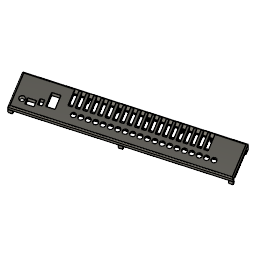
HV Interlock panel (Autodesk Fusion 360 design; units mm, degrees)
Autodesk Fusion 360 part; units mm, degrees
sketch "Sketch1" plane through (0, 0, 0) normal (0, 0, 1) x (1, 0, 0)
  line L0 (152.4, -27.305) -> (-152.4, -27.305)
  line L1 (-152.4, -27.305) -> (-152.4, 27.305)
  line L2 (-152.4, 27.305) -> (152.4, 27.305)
  line L3 (152.4, 27.305) -> (152.4, -27.305)
  line L4 (152.4, -27.305) -> (-152.4, 27.305) construction
  line L5 (-152.4, -27.305) -> (152.4, 27.305) construction
  dimension "d1" = 304.8
  dimension "d2" = 54.61
  constraint horizontal L0
  constraint perpendicular L0 L1
  constraint parallel L0 L2
  constraint parallel L1 L3
  constraint coincident L4 origin
  constraint coincident L5 origin
  measures "d1" distance of L1.end L2.end
  measures "d2" distance of L0.end L1.end
extrude "Extrude1" add sketch "Sketch1" along normal blind 8.001 makes body 1
sketch "Sketch2" plane through (0, 0, 0) normal (0, 0, -1) x (1, 0, 0)
  line L0 (-152.4, -27.305) -> (152.4, -27.305)
  line L1 (152.4, -27.305) -> (152.4, 27.305)
  line L2 (152.4, 27.305) -> (-152.4, 27.305)
  line L3 (-152.4, 27.305) -> (-152.4, -27.305)
  line L4 (152.4, -22.225) -> (-152.4, -22.225)
  line L5 (-152.4, -22.225) -> (-152.4, 22.225)
  line L6 (-152.4, 22.225) -> (152.4, 22.225)
  line L7 (152.4, 22.225) -> (152.4, -22.225)
  line L8 (152.4, -22.225) -> (-152.4, 22.225) construction
  line L9 (-152.4, -22.225) -> (152.4, 22.225) construction
  line L10 (-152.4, 27.305) -> (-146.05, 27.305)
  line L11 (-146.05, 27.305) -> (-146.05, 19.685)
  line L12 (-146.05, 19.685) -> (-152.4, 19.685)
  line L13 (-152.4, 19.685) -> (-152.4, 27.305)
  dimension "d5" = 304.8
  dimension "d6" = 44.45
  dimension "d7" = 6.35
  dimension "d8" = 7.62
  constraint horizontal L4
  constraint perpendicular L4 L5
  constraint parallel L4 L6
  constraint parallel L5 L7
  constraint coincident L8 origin
  constraint coincident L9 origin
  constraint horizontal L10
  constraint vertical L11
  constraint horizontal L12
  constraint vertical L13
  constraint coincident L2.end L3.start
  measures "d5" distance of L5.end L6.end
  measures "d6" distance of L4.end L5.end
  measures "d7" distance of L2.end L10.end
  measures "d8" distance of L2.end L12.end
extrude "Extrude2" add sketch "Sketch2" along normal blind 7.874 contours L3 L5 L6 L11 L12 L13 | L2 L3 L6 L10 L11 L13 bodies 1
pattern_linear "R-Pattern1" count 8 spacing 42.6357 along (1, 0, 0) of "Extrude2"
sketch "Sketch3" plane through (152.4, 0, 0) normal (1, 0, 0) x (0, 1, 0)
  line L0 (-19.685, 0) -> (27.305, 0)
  line L1 (27.305, 0) -> (27.305, 8.001)
  line L2 (27.305, 8.001) -> (-27.305, 8.001)
  line L3 (-27.305, 8.001) -> (-27.305, -7.874)
  line L4 (-27.305, -7.874) -> (-19.685, -7.874)
  line L5 (-19.685, -7.874) -> (-19.685, 0)
  line L6 (-19.685, 0) -> (-22.225, 0)
  line L7 (-22.225, 0) -> (-22.225, -1.6256)
  line L8 (-22.225, -1.6256) -> (-19.685, -1.6256)
  line L9 (-19.685, -1.6256) -> (-19.685, 0)
  dimension "d15" = 2.54
  dimension "d16" = 1.6256
  constraint horizontal L6
  constraint vertical L7
  constraint horizontal L8
  constraint vertical L9
  constraint coincident L0.start L5.end
  measures "d15" distance of L0.start L6.end
  measures "d16" distance of L0.start L8.end
extrude "Extrude3" cut sketch "Sketch3" against normal blind 358.14 contours L5 L6 L7 L8 L9 bodies 1
sketch "Sketch4" plane through (0, 0, 0) normal (0, 0, -1) x (1, 0, 0)
  line L0 (146.05, 22.225) -> (146.05, 27.305)
  line L1 (146.05, 27.305) -> (109.7643, 27.305)
  line L2 (109.7643, 27.305) -> (109.7643, 22.225)
  line L3 (109.7643, 22.225) -> (103.4143, 22.225)
  line L4 (103.4143, 22.225) -> (103.4143, 27.305)
  line L5 (103.4143, 27.305) -> (67.1286, 27.305)
  line L6 (67.1286, 27.305) -> (67.1286, 22.225)
  line L7 (67.1286, 22.225) -> (60.7786, 22.225)
  line L8 (60.7786, 22.225) -> (60.7786, 27.305)
  line L9 (60.7786, 27.305) -> (24.4929, 27.305)
  line L10 (24.4929, 27.305) -> (24.4929, 22.225)
  line L11 (24.4929, 22.225) -> (18.1429, 22.225)
  line L12 (18.1429, 22.225) -> (18.1429, 27.305)
  line L13 (18.1429, 27.305) -> (-18.1429, 27.305)
  line L14 (-18.1429, 27.305) -> (-18.1429, 22.225)
  line L15 (-18.1429, 22.225) -> (-24.4929, 22.225)
  line L16 (-24.4929, 22.225) -> (-24.4929, 27.305)
  line L17 (-24.4929, 27.305) -> (-60.7786, 27.305)
  line L18 (-60.7786, 27.305) -> (-60.7786, 22.225)
  line L19 (-60.7786, 22.225) -> (-67.1286, 22.225)
  line L20 (-67.1286, 22.225) -> (-67.1286, 27.305)
  line L21 (-67.1286, 27.305) -> (-103.4143, 27.305)
  line L22 (-103.4143, 27.305) -> (-103.4143, 22.225)
  line L23 (-103.4143, 22.225) -> (-109.7643, 22.225)
  line L24 (-109.7643, 22.225) -> (-109.7643, 27.305)
  line L25 (-109.7643, 27.305) -> (-146.05, 27.305)
  line L26 (-146.05, 27.305) -> (-146.05, 22.225)
  line L27 (-146.05, 22.225) -> (-152.4, 22.225)
  line L28 (-152.4, 22.225) -> (-152.4, -27.305)
  line L29 (-152.4, -27.305) -> (152.4, -27.305)
  line L30 (152.4, -27.305) -> (152.4, 22.225)
  line L31 (152.4, 22.225) -> (146.05, 22.225)
  line L32 (-152.4, -27.305) -> (-146.05, -27.305)
  line L33 (-146.05, -27.305) -> (-146.05, -22.098)
  line L34 (-146.05, -22.098) -> (-152.4, -22.098)
  line L35 (-152.4, -22.098) -> (-152.4, -27.305)
  dimension "d19" = 6.35
  dimension "d20" = 5.207
  constraint horizontal L32
  constraint vertical L33
  constraint horizontal L34
  constraint vertical L35
  constraint coincident L28.end L29.start
  measures "d19" distance of L28.end L32.end
  measures "d20" distance of L28.end L34.end
extrude "Extrude4" add sketch "Sketch4" along normal up to surface (7.874 mm away) separate body contours L28 L29 L32 L33 L34 L35 makes body 2
pattern_linear "R-Pattern2" count 3 spacing 149.225 along (1, 0, 0) of "Extrude4" makes body 3 makes body 4
sketch "Sketch5" plane through (-152.4, 0, 0) normal (-1, 0, 0) x (0, -1, 0)
  line L0 (-27.305, -7.874) -> (-22.098, -7.874)
  line L1 (-22.098, -7.874) -> (-22.098, 0)
  line L2 (-22.098, 0) -> (-27.305, 0)
  line L3 (-27.305, 0) -> (-27.305, -7.874)
  line L4 (-24.638, 0) -> (-24.638, -1.524)
  line L5 (-24.638, -1.524) -> (-22.098, -3.937)
  line L6 (-22.098, -3.937) -> (-24.7015, -7.874)
  line L7 (-24.7015, -7.874) -> (-22.098, -7.874)
  line L8 (-22.098, -7.874) -> (-22.098, 0)
  line L9 (-22.098, 0) -> (-24.638, 0)
  point P0 (-24.638, 0)
  dimension "d27" = 2.54
  dimension "d28" = 1.524
  constraint coincident L2 P0
  constraint coincident P0 L4.start
  constraint perpendicular L2 L4
  constraint midpoint L1 L5.end
  constraint midpoint L0 L6.end
  constraint coincident L0.end L1.start
  constraint coincident L1.end L2.start
  measures "d27" distance of L1 P0
  measures "d28" distance of P0 L4.end
extrude "Extrude5" cut sketch "Sketch5" against normal blind 358.14 contours L0 L1 L6 L7 L8 | L1 L2 L4 L5 L8 L9 bodies 2 3 4
sketch "Sketch6" plane through (-152.4, 0, 0) normal (-1, 0, 0) x (0, -1, 0)
  line L0 (22.225, -1.6256) -> (19.685, -1.6256)
  line L1 (19.685, -1.6256) -> (19.685, -7.874)
  line L2 (19.685, -7.874) -> (27.305, -7.874)
  line L3 (27.305, -7.874) -> (27.305, 8.001)
  line L4 (27.305, 8.001) -> (-27.305, 8.001)
  line L5 (-27.305, 8.001) -> (-27.305, 0)
  line L6 (-27.305, 0) -> (22.225, 0)
  line L7 (22.225, 0) -> (22.225, -1.6256)
  line L8 (-24.6876, 0) -> (-24.6876, 4.0005)
  line L9 (-24.6876, 4.0005) -> (-21.59, 4.0005)
  line L10 (-21.59, 4.0005) -> (-21.59, 0)
  line L11 (-21.59, 0) -> (-24.6876, 0)
  constraint coincident L6 L8.start
  constraint perpendicular L4 L8
  constraint perpendicular L8 L9
  constraint coincident L6 L10.end
  constraint perpendicular L6 L10
extrude "Extrude6" cut sketch "Sketch6" against normal blind 320.04 contours L6 L8 L9 L10 L11 bodies 1
fillet "Fillet1" radius 1.27 1 edges at (0, 24.6876, 4.0005) on bodies 1
sketch "Sketch8" plane through (0, 0, 8.001) normal (0, 0, 1) x (-1, 0, 0)
  line L0 (-152.4, -27.305) -> (152.4, -27.305)
  line L1 (152.4, -27.305) -> (152.4, 27.305)
  line L2 (152.4, 27.305) -> (-152.4, 27.305)
  line L3 (-152.4, 27.305) -> (-152.4, -27.305)
  line L4 (2.794, 5.715) -> (-2.794, 5.715)
  line L5 (-2.794, 5.715) -> (-2.794, 20.955)
  line L6 (-2.794, 20.955) -> (2.794, 20.955)
  line L7 (2.794, 20.955) -> (2.794, 5.715)
  line L8 (2.794, 5.715) -> (-2.794, 20.955) construction
  line L9 (-2.794, 5.715) -> (2.794, 20.955) construction
  point P0 (0, 13.335)
  dimension "d35" = 5.588
  dimension "d36" = 15.24
  dimension "d37" = 13.97
  constraint horizontal L4
  constraint perpendicular L4 L5
  constraint parallel L4 L6
  constraint parallel L5 L7
  constraint coincident L8 P0
  constraint coincident L9 P0
  measures "d35" distance of L5.end L6.end
  measures "d36" distance of L4.end L5.end
  measures "d37" distance of L2 P0
sketch "PCB" plane through (0, 0, 8.001) normal (0, 0, 1) x (-1, 0, 0)
  line L0 (-152.4, -27.305) -> (152.4, -27.305)
  line L1 (152.4, -27.305) -> (152.4, 27.305)
  line L2 (152.4, 27.305) -> (-152.4, 27.305)
  line L3 (-152.4, 27.305) -> (-152.4, -27.305)
  circle A0 centre (-32.5558, -7.8785) radius 0.85
  circle A1 centre (-37.4758, -7.8785) radius 0.85
  circle A2 centre (-139.3358, -10.4185) radius 0.6
  circle A3 centre (32.5242, -7.8785) radius 0.85
  circle A4 centre (22.5242, -7.8785) radius 0.85
  circle A5 centre (-136.7958, -7.8785) radius 0.85
  circle A6 centre (-100.0708, 3.8415) radius 0.5
  circle A7 centre (27.4442, -12.9585) radius 0.85
  circle A8 centre (29.9842, -10.4185) radius 0.6
  circle A9 centre (-129.8408, -10.4185) radius 0.5
  circle A10 centre (-102.6108, 3.8415) radius 0.5
  circle A11 centre (17.4442, -12.9585) radius 0.85
  circle A12 centre (-141.8758, -7.8785) radius 0.85
  circle A13 centre (42.5242, -7.8785) radius 0.85
  circle A14 centre (-27.4758, -7.8785) radius 0.85
  circle A15 centre (19.9842, -10.4185) radius 0.6
  circle A16 centre (-113.6508, -4.6785) radius 0.5
  circle A17 centre (-222.1058, -16.0685) radius 3.2
  circle A18 centre (37.4442, -7.8785) radius 0.85
  circle A19 centre (-141.8758, -12.9585) radius 0.85
  circle A20 centre (-42.5558, -7.8785) radius 0.85
  circle A21 centre (-124.6058, -12.9585) radius 0.5
  circle A22 centre (-129.8408, -12.9585) radius 0.5
  circle A23 centre (-124.6058, -10.4185) radius 0.5
  circle A24 centre (-40.0158, -10.4185) radius 0.6
  circle A25 centre (-30.0158, -10.4185) radius 0.6
  circle A26 centre (-42.5558, -12.9585) radius 0.85
  circle A27 centre (-37.4758, -12.9585) radius 0.85
  circle A28 centre (39.9842, -10.4185) radius 0.6
  circle A29 centre (-136.7958, -12.9585) radius 0.85
  circle A30 centre (27.4442, -7.8785) radius 0.85
  circle A31 centre (-103.6256, -4.568) radius 0.7
  circle A32 centre (-78.4158, 15.6015) radius 0.5
  circle A33 centre (-116.1908, -4.6785) radius 0.5
  circle A34 centre (-98.5456, -4.568) radius 0.7
  circle A35 centre (-32.5558, -12.9585) radius 0.85
  circle A36 centre (-49.9558, -10.4185) radius 0.6
  circle A37 centre (-58.4158, 10.6015) radius 0.5
  circle A38 centre (-68.4158, 13.1015) radius 0.5
  circle A39 centre (-68.4158, 10.6015) radius 0.5
  circle A40 centre (-57.4758, -7.8785) radius 0.85
  circle A41 centre (-68.4158, 15.6015) radius 0.5
  circle A42 centre (-67.4758, -7.8785) radius 0.85
  circle A43 centre (-72.5558, -7.8785) radius 0.85
  circle A44 centre (-47.4158, -7.8785) radius 0.85
  circle A45 centre (-58.4158, 15.6015) radius 0.5
  circle A46 centre (-52.4958, -7.8785) radius 0.85
  circle A47 centre (-78.4158, 13.1015) radius 0.5
  circle A48 centre (-70.0158, -10.4185) radius 0.6
  circle A49 centre (-67.4758, -12.9585) radius 0.85
  circle A50 centre (-57.4758, -12.9585) radius 0.85
  circle A51 centre (-48.4158, 10.6015) radius 0.5
  circle A52 centre (-27.4758, -12.9585) radius 0.85
  circle A53 centre (-48.4158, 15.6015) radius 0.5
  circle A54 centre (-78.4158, 10.6015) radius 0.5
  circle A55 centre (-58.4158, 13.1015) radius 0.5
  circle A56 centre (-62.5558, -7.8785) radius 0.85
  circle A57 centre (-48.4158, 13.1015) radius 0.5
  circle A58 centre (-60.0158, -10.4185) radius 0.6
  circle A59 centre (-72.5558, -12.9585) radius 0.85
  circle A60 centre (-62.5558, -12.9585) radius 0.85
  circle A61 centre (-47.4158, -12.9585) radius 0.85
  circle A62 centre (-52.4958, -12.9585) radius 0.85
  circle A63 centre (-10.0158, -10.4185) radius 0.6
  circle A64 centre (17.4442, -7.8785) radius 0.85
  circle A65 centre (-7.4758, -7.8785) radius 0.85
  circle A66 centre (-17.4758, -7.8785) radius 0.85
  line L4 (-230.9558, 22.6815) -> (-230.9558, -21.7685)
  circle A67 centre (-20.0158, -10.4185) radius 0.6
  circle A68 centre (32.5242, -12.9585) radius 0.85
  circle A69 centre (-7.4758, -12.9585) radius 0.85
  circle A70 centre (-12.5558, -12.9585) radius 0.85
  circle A71 centre (42.5242, -12.9585) radius 0.85
  circle A72 centre (-22.5558, -12.9585) radius 0.85
  circle A73 centre (37.4442, -12.9585) radius 0.85
  circle A74 centre (22.5242, -12.9585) radius 0.85
  circle A75 centre (-17.4758, -12.9585) radius 0.85
  circle A76 centre (97.4442, -7.8785) radius 0.85
  circle A77 centre (7.4442, -7.8785) radius 0.85
  circle A78 centre (-18.4158, 10.6015) radius 0.5
  circle A79 centre (72.5242, -12.9585) radius 0.85
  circle A80 centre (117.4442, -7.8785) radius 0.85
  circle A81 centre (62.5242, -12.9585) radius 0.85
  circle A82 centre (-2.5558, -12.9585) radius 0.85
  circle A83 centre (-28.4158, 10.6015) radius 0.5
  circle A84 centre (87.4442, -12.9585) radius 0.85
  circle A85 centre (77.2442, 10.4015) radius 0.5
  circle A86 centre (57.4442, -12.9585) radius 0.85
  circle A87 centre (77.2442, 12.9015) radius 0.5
  circle A88 centre (122.5242, -7.8785) radius 0.85
  circle A89 centre (1.5842, 10.6015) radius 0.5
  circle A90 centre (-2.5558, -7.8785) radius 0.85
  circle A91 centre (62.5242, -7.8785) radius 0.85
  circle A92 centre (86.6242, 12.9015) radius 0.5
  circle A93 centre (67.8642, 12.9015) radius 0.5
  circle A94 centre (20.9642, 12.9015) radius 0.5
  circle A95 centre (11.5842, 13.1015) radius 0.5
  circle A96 centre (30.3442, 12.9015) radius 0.5
  circle A97 centre (49.1042, 10.4015) radius 0.5
  circle A98 centre (39.7242, 12.9015) radius 0.5
  circle A99 centre (58.4842, 10.4015) radius 0.5
  circle A100 centre (67.8642, 10.4015) radius 0.5
  circle A101 centre (30.3442, 10.4015) radius 0.5
  circle A102 centre (47.4442, -12.9585) radius 0.85
  circle A103 centre (30.3442, 15.4015) radius 0.5
  circle A104 centre (20.9642, 10.4015) radius 0.5
  circle A105 centre (107.4442, -7.8785) radius 0.85
  circle A106 centre (49.1042, 12.9015) radius 0.5
  circle A107 centre (-8.4158, 10.6015) radius 0.5
  circle A108 centre (112.5242, -7.8785) radius 0.85
  circle A109 centre (92.5242, -7.8785) radius 0.85
  circle A110 centre (58.4842, 12.9015) radius 0.5
  circle A111 centre (11.5842, 15.6015) radius 0.5
  circle A112 centre (11.5842, 10.6015) radius 0.5
  circle A113 centre (59.9842, -10.4185) radius 0.6
  circle A114 centre (49.9842, -10.4185) radius 0.6
  circle A115 centre (39.7242, 15.4015) radius 0.5
  circle A116 centre (2.5242, -7.8785) radius 0.85
  circle A117 centre (-0.0158, -10.4185) radius 0.6
  circle A118 centre (82.5242, -12.9585) radius 0.85
  circle A119 centre (52.5242, -12.9585) radius 0.85
  circle A120 centre (-38.4158, 10.6015) radius 0.5
  circle A121 centre (77.4442, -12.9585) radius 0.85
  circle A122 centre (-8.4158, 13.1015) radius 0.5
  circle A123 centre (9.9842, -10.4185) radius 0.6
  circle A124 centre (20.9642, 15.4015) radius 0.5
  circle A125 centre (69.9842, -10.4185) radius 0.6
  circle A126 centre (86.6242, 10.4015) radius 0.5
  circle A127 centre (-18.4158, 13.1015) radius 0.5
  circle A128 centre (89.9842, -10.4185) radius 0.6
  circle A129 centre (-18.4158, 15.6015) radius 0.5
  circle A130 centre (97.4442, -12.9585) radius 0.85
  circle A131 centre (-222.1058, 15.9315) radius 3.2
  circle A132 centre (77.4442, -7.8785) radius 0.85
  circle A133 centre (92.5242, -12.9585) radius 0.85
  circle A134 centre (-12.5558, -7.8785) radius 0.85
  circle A135 centre (82.5242, -7.8785) radius 0.85
  circle A136 centre (112.5242, -12.9585) radius 0.85
  circle A137 centre (122.5242, -12.9585) radius 0.85
  circle A138 centre (-8.4158, 15.6015) radius 0.5
  circle A139 centre (-28.4158, 15.6015) radius 0.5
  circle A140 centre (-38.4158, 15.6015) radius 0.5
  circle A141 centre (67.4442, -12.9585) radius 0.85
  circle A142 centre (117.4442, -12.9585) radius 0.85
  circle A143 centre (102.5242, -12.9585) radius 0.85
  circle A144 centre (2.5242, -12.9585) radius 0.85
  circle A145 centre (119.9842, -10.4185) radius 0.6
  circle A146 centre (12.5242, -12.9585) radius 0.85
  circle A147 centre (109.9842, -10.4185) radius 0.6
  circle A148 centre (107.4442, -12.9585) radius 0.85
  circle A149 centre (7.4442, -12.9585) radius 0.85
  circle A150 centre (79.9842, -10.4185) radius 0.6
  circle A151 centre (12.5242, -7.8785) radius 0.85
  circle A152 centre (-28.4158, 13.1015) radius 0.5
  circle A153 centre (87.4442, -7.8785) radius 0.85
  circle A154 centre (-38.4158, 13.1015) radius 0.5
  circle A155 centre (99.9842, -10.4185) radius 0.6
  circle A156 centre (-22.5558, -7.8785) radius 0.85
  circle A157 centre (72.5242, -7.8785) radius 0.85
  circle A158 centre (49.1042, 15.4015) radius 0.5
  circle A159 centre (105.3842, 12.9015) radius 0.5
  circle A160 centre (67.4442, -7.8785) radius 0.85
  circle A161 centre (105.3842, 15.4015) radius 0.5
  line L5 (251.6442, 22.6815) -> (-230.9558, 22.6815)
  circle A162 centre (47.4442, -7.8785) radius 0.85
  line L6 (251.6442, -21.7685) -> (251.6442, 22.6815)
  line L7 (-230.9558, -21.7685) -> (251.6442, -21.7685)
  circle A163 centre (96.0042, 15.4015) radius 0.5
  circle A164 centre (242.8942, 15.9315) radius 3.2
  circle A165 centre (52.5242, -7.8785) radius 0.85
  circle A166 centre (242.8942, -16.0685) radius 3.2
  circle A167 centre (96.0042, 12.9015) radius 0.5
  circle A168 centre (102.5242, -7.8785) radius 0.85
  circle A169 centre (77.2442, 15.4015) radius 0.5
  circle A170 centre (1.5842, 15.6015) radius 0.5
  circle A171 centre (58.4842, 15.4015) radius 0.5
  circle A172 centre (105.3842, 10.4015) radius 0.5
  circle A173 centre (39.7242, 10.4015) radius 0.5
  circle A174 centre (1.5842, 13.1015) radius 0.5
  circle A175 centre (86.6242, 15.4015) radius 0.5
  circle A176 centre (67.8642, 15.4015) radius 0.5
  circle A177 centre (57.4442, -7.8785) radius 0.85
  circle A178 centre (96.0042, 10.4015) radius 0.5
sketch "Sketch11" plane through (0, 0, 8.001) normal (0, 0, 1) x (1, 0, 0)
sketch "Sketch12" plane through (0, 0, 0) normal (0, 0, -1) x (1, 0, 0)
  line L0 (-152.4, -21.59) -> (152.4, -21.59)
  line L1 (152.4, -21.59) -> (152.4, 22.225)
  line L2 (152.4, 22.225) -> (146.05, 22.225)
  line L3 (146.05, 22.225) -> (146.05, 27.305)
  line L4 (146.05, 27.305) -> (109.7643, 27.305)
  line L5 (109.7643, 27.305) -> (109.7643, 22.225)
  line L6 (109.7643, 22.225) -> (103.4143, 22.225)
  line L7 (103.4143, 22.225) -> (103.4143, 27.305)
  line L8 (103.4143, 27.305) -> (67.1286, 27.305)
  line L9 (67.1286, 27.305) -> (67.1286, 22.225)
  line L10 (67.1286, 22.225) -> (60.7786, 22.225)
  line L11 (60.7786, 22.225) -> (60.7786, 27.305)
  line L12 (60.7786, 27.305) -> (24.4929, 27.305)
  line L13 (24.4929, 27.305) -> (24.4929, 22.225)
  line L14 (24.4929, 22.225) -> (18.1429, 22.225)
  line L15 (18.1429, 22.225) -> (18.1429, 27.305)
  line L16 (18.1429, 27.305) -> (-18.1429, 27.305)
  line L17 (-18.1429, 27.305) -> (-18.1429, 22.225)
  line L18 (-18.1429, 22.225) -> (-24.4929, 22.225)
  line L19 (-24.4929, 22.225) -> (-24.4929, 27.305)
  line L20 (-24.4929, 27.305) -> (-60.7786, 27.305)
  line L21 (-60.7786, 27.305) -> (-60.7786, 22.225)
  line L22 (-60.7786, 22.225) -> (-67.1286, 22.225)
  line L23 (-67.1286, 22.225) -> (-67.1286, 27.305)
  line L24 (-67.1286, 27.305) -> (-103.4143, 27.305)
  line L25 (-103.4143, 27.305) -> (-103.4143, 22.225)
  line L26 (-103.4143, 22.225) -> (-109.7643, 22.225)
  line L27 (-109.7643, 22.225) -> (-109.7643, 27.305)
  line L28 (-109.7643, 27.305) -> (-146.05, 27.305)
  line L29 (-146.05, 27.305) -> (-146.05, 22.225)
  line L30 (-146.05, 22.225) -> (-152.4, 22.225)
  line L31 (-152.4, 22.225) -> (-152.4, -21.59)
  line L32 (-127, -15.24) -> (81.28, -15.24)
  line L33 (81.28, -15.24) -> (81.28, -5.08)
  line L34 (81.28, -5.08) -> (-127, -5.08)
  line L35 (-127, -5.08) -> (-127, -15.24)
  constraint horizontal L32
  constraint vertical L33
  constraint horizontal L34
  constraint vertical L35
extrude "Extrude9" cut sketch "Sketch12" against normal blind 4.699 contours L32 L33 L34 L35 bodies 1
sketch "Sketch13" plane through (0, 0, 8.001) normal (0, 0, 1) x (-1, 0, 0)
  line L0 (-152.4, -27.305) -> (152.4, -27.305)
  line L1 (152.4, -27.305) -> (152.4, 27.305)
  line L2 (152.4, 27.305) -> (-152.4, 27.305)
  line L3 (-152.4, 27.305) -> (-152.4, -27.305)
  circle A0 centre (-69.977, -10.414) radius 3.81
  dimension "d58" = 7.62
  measures "d58" diameter of A0
extrude "Extrude10" cut sketch "Sketch13" against normal blind 33.02 contours A0 bodies 1
pattern_linear "R-Pattern5" count 20 spacing 10.0076 along (-1, 0, 0) of "Extrude10"
sketch "Sketch14" plane through (0, 0, 8.001) normal (0, 0, 1) x (-1, 0, 0)
  circle A0 centre (120.1674, -10.414) radius 3.81
  circle A1 centre (110.1598, -10.414) radius 3.81
  circle A2 centre (100.1522, -10.414) radius 3.81
  circle A3 centre (90.1446, -10.414) radius 3.81
  circle A4 centre (80.137, -10.414) radius 3.81
  circle A5 centre (70.1294, -10.414) radius 3.81
  circle A6 centre (60.1218, -10.414) radius 3.81
  circle A7 centre (50.1142, -10.414) radius 3.81
  circle A8 centre (40.1066, -10.414) radius 3.81
  circle A9 centre (30.099, -10.414) radius 3.81
  circle A10 centre (20.0914, -10.414) radius 3.81
  circle A11 centre (10.0838, -10.414) radius 3.81
  circle A12 centre (0.0762, -10.414) radius 3.81
  circle A13 centre (-9.9314, -10.414) radius 3.81
  circle A14 centre (-19.939, -10.414) radius 3.81
  circle A15 centre (-29.9466, -10.414) radius 3.81
  circle A16 centre (-39.9542, -10.414) radius 3.81
  circle A17 centre (-49.9618, -10.414) radius 3.81
  circle A18 centre (-59.9694, -10.414) radius 3.81
  circle A19 centre (-69.977, -10.414) radius 3.81
  line L0 (-152.4, -27.305) -> (152.4, -27.305)
  line L1 (152.4, -27.305) -> (152.4, 27.305)
  line L2 (152.4, 27.305) -> (-152.4, 27.305)
  line L3 (-152.4, 27.305) -> (-152.4, -27.305)
  circle A20 centre (-139.446, -10.414) radius 4.191
  line L4 (-121.1105, -16.5252) -> (-133.3735, -16.5252)
  line L5 (-133.3735, -16.5252) -> (-133.3735, -7.0652)
  line L6 (-133.3735, -7.0652) -> (-121.1105, -7.0652)
  line L7 (-121.1105, -7.0652) -> (-121.1105, -16.5252)
  line L8 (-121.1105, -16.5252) -> (-133.3735, -7.0652) construction
  line L9 (-133.3735, -16.5252) -> (-121.1105, -7.0652) construction
  line L10 (-117.6944, -2.6856) -> (-111.7381, -2.6856)
  line L11 (-111.7381, -2.6856) -> (-111.7381, -11.8828)
  line L12 (-111.7381, -11.8828) -> (-117.6944, -11.8828)
  line L13 (-117.6944, -11.8828) -> (-117.6944, -2.6856)
  line L14 (-94.7413, -10.795) -> (-107.1873, -10.795)
  line L15 (-107.1873, -10.795) -> (-107.1873, 10.795)
  line L16 (-107.1873, 10.795) -> (-94.7413, 10.795)
  line L17 (-94.7413, 10.795) -> (-94.7413, -10.795)
  line L18 (-94.7413, -10.795) -> (-107.1873, 10.795) construction
  line L19 (-107.1873, -10.795) -> (-94.7413, 10.795) construction
  point P0 (-127.242, -11.7952)
  point P1 (-100.9643, 0)
  dimension "d65" = 8.382
  dimension "d66" = 12.446
  dimension "d67" = 21.59
  constraint horizontal L4
  constraint perpendicular L4 L5
  constraint parallel L4 L6
  constraint parallel L5 L7
  constraint coincident L8 P0
  constraint coincident L9 P0
  constraint horizontal L10
  constraint vertical L11
  constraint horizontal L12
  constraint vertical L13
  constraint horizontal L14
  constraint perpendicular L14 L15
  constraint parallel L14 L16
  constraint parallel L15 L17
  constraint coincident L18 P1
  constraint coincident L19 P1
  measures "d65" diameter of A20
  measures "d66" distance of L15.end L16.end
  measures "d67" distance of L14.end L15.end
extrude "Extrude11" cut sketch "Sketch14" against normal blind 22.86 contours A20 | L4 L5 L6 L7 | L10 L11 L12 L13 | L14 L15 L16 L17 bodies 1
sketch "Sketch15" plane through (0, 0, 0) normal (0, 0, -1) x (1, 0, 0)
  line L0 (133.3735, -7.0652) -> (133.3735, -16.5252)
  line L1 (133.3735, -16.5252) -> (121.1105, -16.5252)
  line L2 (121.1105, -16.5252) -> (121.1105, -7.0652)
  line L3 (121.1105, -7.0652) -> (133.3735, -7.0652)
  line L4 (111.7381, -11.8828) -> (111.7381, -2.6856)
  line L5 (111.7381, -2.6856) -> (117.6944, -2.6856)
  line L6 (117.6944, -2.6856) -> (117.6944, -11.8828)
  line L7 (117.6944, -11.8828) -> (111.7381, -11.8828)
  circle A0 centre (139.446, -10.414) radius 4.191
  line L8 (107.1873, 10.795) -> (107.1873, -10.795)
  line L9 (107.1873, -10.795) -> (94.7413, -10.795)
  line L10 (94.7413, -10.795) -> (94.7413, 10.795)
  line L11 (94.7413, 10.795) -> (107.1873, 10.795)
  line L12 (81.28, -15.24) -> (-127, -15.24)
  line L13 (-127, -15.24) -> (-127, -5.08)
  line L14 (-127, -5.08) -> (81.28, -5.08)
  line L15 (81.28, -5.08) -> (81.28, -15.24)
  line L16 (-152.4, -21.59) -> (152.4, -21.59)
  line L17 (152.4, -21.59) -> (152.4, 22.225)
  line L18 (152.4, 22.225) -> (146.05, 22.225)
  line L19 (146.05, 22.225) -> (146.05, 27.305)
  line L20 (146.05, 27.305) -> (109.7643, 27.305)
  line L21 (109.7643, 27.305) -> (109.7643, 22.225)
  line L22 (109.7643, 22.225) -> (103.4143, 22.225)
  line L23 (103.4143, 22.225) -> (103.4143, 27.305)
  line L24 (103.4143, 27.305) -> (67.1286, 27.305)
  line L25 (67.1286, 27.305) -> (67.1286, 22.225)
  line L26 (67.1286, 22.225) -> (60.7786, 22.225)
  line L27 (60.7786, 22.225) -> (60.7786, 27.305)
  line L28 (60.7786, 27.305) -> (24.4929, 27.305)
  line L29 (24.4929, 27.305) -> (24.4929, 22.225)
  line L30 (24.4929, 22.225) -> (18.1429, 22.225)
  line L31 (18.1429, 22.225) -> (18.1429, 27.305)
  line L32 (18.1429, 27.305) -> (-18.1429, 27.305)
  line L33 (-18.1429, 27.305) -> (-18.1429, 22.225)
  line L34 (-18.1429, 22.225) -> (-24.4929, 22.225)
  line L35 (-24.4929, 22.225) -> (-24.4929, 27.305)
  line L36 (-24.4929, 27.305) -> (-60.7786, 27.305)
  line L37 (-60.7786, 27.305) -> (-60.7786, 22.225)
  line L38 (-60.7786, 22.225) -> (-67.1286, 22.225)
  line L39 (-67.1286, 22.225) -> (-67.1286, 27.305)
  line L40 (-67.1286, 27.305) -> (-103.4143, 27.305)
  line L41 (-103.4143, 27.305) -> (-103.4143, 22.225)
  line L42 (-103.4143, 22.225) -> (-109.7643, 22.225)
  line L43 (-109.7643, 22.225) -> (-109.7643, 27.305)
  line L44 (-109.7643, 27.305) -> (-146.05, 27.305)
  line L45 (-146.05, 27.305) -> (-146.05, 22.225)
  line L46 (-146.05, 22.225) -> (-152.4, 22.225)
  line L47 (-152.4, 22.225) -> (-152.4, -21.59)
  line L48 (133.858, -5.08) -> (145.034, -5.08)
  line L49 (145.034, -5.08) -> (145.034, -15.748)
  line L50 (145.034, -15.748) -> (133.858, -15.748)
  line L51 (133.858, -15.748) -> (133.858, -5.08)
  line L52 (133.858, -5.08) -> (145.034, -15.748) construction
  line L53 (145.034, -5.08) -> (133.858, -15.748) construction
  point P0 (139.446, -10.414)
  dimension "d70" = 11.176
  dimension "d71" = 10.668
  constraint horizontal L48
  constraint perpendicular L48 L49
  constraint parallel L48 L50
  constraint parallel L49 L51
  constraint coincident L52 P0
  constraint coincident L53 P0
  constraint coincident P0 A0.centre
  measures "d70" distance of L49.end L50.end
  measures "d71" distance of L48.end L49.end
sketch "Sketch16" plane through (0, 0, 8.001) normal (0, 0, 1) x (-1, 0, 0)
  line L0 (-133.3735, -16.5252) -> (-133.3735, -7.0652)
  line L1 (-133.3735, -7.0652) -> (-121.1105, -7.0652)
  line L2 (-121.1105, -7.0652) -> (-121.1105, -16.5252)
  line L3 (-121.1105, -16.5252) -> (-133.3735, -16.5252)
  line L4 (-111.7381, -2.6856) -> (-111.7381, -11.8828)
  line L5 (-111.7381, -11.8828) -> (-117.6944, -11.8828)
  line L6 (-117.6944, -11.8828) -> (-117.6944, -2.6856)
  line L7 (-117.6944, -2.6856) -> (-111.7381, -2.6856)
  circle A0 centre (-139.446, -10.414) radius 4.191
  line L8 (-107.1873, -10.795) -> (-107.1873, 10.795)
  line L9 (-107.1873, 10.795) -> (-94.7413, 10.795)
  line L10 (-94.7413, 10.795) -> (-94.7413, -10.795)
  line L11 (-94.7413, -10.795) -> (-107.1873, -10.795)
  circle A1 centre (120.1674, -10.414) radius 3.81
  circle A2 centre (110.1598, -10.414) radius 3.81
  circle A3 centre (100.1522, -10.414) radius 3.81
  circle A4 centre (90.1446, -10.414) radius 3.81
  circle A5 centre (80.137, -10.414) radius 3.81
  circle A6 centre (70.1294, -10.414) radius 3.81
  circle A7 centre (60.1218, -10.414) radius 3.81
  circle A8 centre (50.1142, -10.414) radius 3.81
  circle A9 centre (40.1066, -10.414) radius 3.81
  circle A10 centre (30.099, -10.414) radius 3.81
  circle A11 centre (20.0914, -10.414) radius 3.81
  circle A12 centre (10.0838, -10.414) radius 3.81
  circle A13 centre (0.0762, -10.414) radius 3.81
  circle A14 centre (-9.9314, -10.414) radius 3.81
  circle A15 centre (-19.939, -10.414) radius 3.81
  circle A16 centre (-29.9466, -10.414) radius 3.81
  circle A17 centre (-39.9542, -10.414) radius 3.81
  circle A18 centre (-49.9618, -10.414) radius 3.81
  circle A19 centre (-59.9694, -10.414) radius 3.81
  circle A20 centre (-69.977, -10.414) radius 3.81
  line L12 (-152.4, -27.305) -> (152.4, -27.305)
  line L13 (152.4, -27.305) -> (152.4, 27.305)
  line L14 (152.4, 27.305) -> (-152.4, 27.305)
  line L15 (-152.4, 27.305) -> (-152.4, -27.305)
  line L16 (-5.5489, 4.8134) -> (-11.3909, 4.8134)
  line L17 (-11.3909, 4.8134) -> (-11.3909, 21.3234)
  line L18 (-11.3909, 21.3234) -> (-5.5489, 21.3234)
  line L19 (-5.5489, 21.3234) -> (-5.5489, 4.8134)
  line L20 (-5.5489, 4.8134) -> (-11.3909, 21.3234) construction
  line L21 (-11.3909, 4.8134) -> (-5.5489, 21.3234) construction
  line L22 (4.4385, 4.9431) -> (-1.4035, 21.4531) construction
  line L23 (4.4385, 21.4531) -> (4.4385, 4.9431)
  line L24 (-1.4035, 4.9431) -> (4.4385, 21.4531) construction
  line L25 (4.4385, 4.9431) -> (-1.4035, 4.9431)
  line L26 (-1.4035, 4.9431) -> (-1.4035, 21.4531)
  line L27 (-1.4035, 21.4531) -> (4.4385, 21.4531)
  line L28 (14.4907, 4.8782) -> (8.6487, 21.3882) construction
  line L29 (14.4907, 21.3882) -> (14.4907, 4.8782)
  line L30 (8.6487, 4.8782) -> (14.4907, 21.3882) construction
  line L31 (14.4907, 4.8782) -> (8.6487, 4.8782)
  line L32 (8.6487, 4.8782) -> (8.6487, 21.3882)
  line L33 (8.6487, 21.3882) -> (14.4907, 21.3882)
  line L34 (-15.4191, 4.8134) -> (-21.2611, 21.3234) construction
  line L35 (-15.4191, 21.3234) -> (-15.4191, 4.8134)
  line L36 (-21.2611, 4.8134) -> (-15.4191, 21.3234) construction
  line L37 (-15.4191, 4.8134) -> (-21.2611, 4.8134)
  line L38 (-21.2611, 4.8134) -> (-21.2611, 21.3234)
  line L39 (-21.2611, 21.3234) -> (-15.4191, 21.3234)
  line L40 (-25.3834, 4.9074) -> (-31.2254, 21.4174) construction
  line L41 (-25.3834, 21.4174) -> (-25.3834, 4.9074)
  line L42 (-31.2254, 4.9074) -> (-25.3834, 21.4174) construction
  line L43 (-25.3834, 4.9074) -> (-31.2254, 4.9074)
  line L44 (-31.2254, 4.9074) -> (-31.2254, 21.4174)
  line L45 (-31.2254, 21.4174) -> (-25.3834, 21.4174)
  line L46 (-35.4715, 4.8488) -> (-41.3135, 21.3588) construction
  line L47 (-35.4715, 21.3588) -> (-35.4715, 4.8488)
  line L48 (-41.3135, 4.8488) -> (-35.4715, 21.3588) construction
  line L49 (-35.4715, 4.8488) -> (-41.3135, 4.8488)
  line L50 (-41.3135, 4.8488) -> (-41.3135, 21.3588)
  line L51 (-41.3135, 21.3588) -> (-35.4715, 21.3588)
  line L52 (-45.4896, 4.8704) -> (-51.3316, 21.3804) construction
  line L53 (-45.4896, 21.3804) -> (-45.4896, 4.8704)
  line L54 (-51.3316, 4.8704) -> (-45.4896, 21.3804) construction
  line L55 (-45.4896, 4.8704) -> (-51.3316, 4.8704)
  line L56 (-51.3316, 4.8704) -> (-51.3316, 21.3804)
  line L57 (-51.3316, 21.3804) -> (-45.4896, 21.3804)
  line L58 (-55.4748, 5.0416) -> (-61.3168, 21.5516) construction
  line L59 (-55.4748, 21.5516) -> (-55.4748, 5.0416)
  line L60 (-61.3168, 5.0416) -> (-55.4748, 21.5516) construction
  line L61 (-55.4748, 5.0416) -> (-61.3168, 5.0416)
  line L62 (-61.3168, 5.0416) -> (-61.3168, 21.5516)
  line L63 (-61.3168, 21.5516) -> (-55.4748, 21.5516)
  line L64 (-65.46, 4.7563) -> (-71.302, 21.2663) construction
  line L65 (-65.46, 21.2663) -> (-65.46, 4.7563)
  line L66 (-71.302, 4.7563) -> (-65.46, 21.2663) construction
  line L67 (-65.46, 4.7563) -> (-71.302, 4.7563)
  line L68 (-71.302, 4.7563) -> (-71.302, 21.2663)
  line L69 (-71.302, 21.2663) -> (-65.46, 21.2663)
  line L70 (-75.3881, 4.8134) -> (-81.2301, 21.3234) construction
  line L71 (-75.3881, 21.3234) -> (-75.3881, 4.8134)
  line L72 (-81.2301, 4.8134) -> (-75.3881, 21.3234) construction
  line L73 (-75.3881, 4.8134) -> (-81.2301, 4.8134)
  line L74 (-81.2301, 4.8134) -> (-81.2301, 21.3234)
  line L75 (-81.2301, 21.3234) -> (-75.3881, 21.3234)
  line L76 (23.9678, 4.7519) -> (18.1258, 21.2619) construction
  line L77 (18.1258, 4.7519) -> (23.9678, 21.2619) construction
  line L78 (23.9678, 21.2619) -> (23.9678, 4.7519)
  line L79 (18.1258, 4.7519) -> (18.1258, 21.2619)
  line L80 (23.9678, 4.7519) -> (18.1258, 4.7519)
  line L81 (18.1258, 21.2619) -> (23.9678, 21.2619)
  line L82 (33.288, 4.8782) -> (27.446, 21.3882) construction
  line L83 (27.446, 4.8782) -> (33.288, 21.3882) construction
  line L84 (33.288, 21.3882) -> (33.288, 4.8782)
  line L85 (27.446, 4.8782) -> (27.446, 21.3882)
  line L86 (33.288, 4.8782) -> (27.446, 4.8782)
  line L87 (27.446, 21.3882) -> (33.288, 21.3882)
  line L88 (42.6059, 4.5623) -> (36.7639, 21.0723) construction
  line L89 (36.7639, 4.5623) -> (42.6059, 21.0723) construction
  line L90 (42.6059, 21.0723) -> (42.6059, 4.5623)
  line L91 (36.7639, 4.5623) -> (36.7639, 21.0723)
  line L92 (42.6059, 4.5623) -> (36.7639, 4.5623)
  line L93 (36.7639, 21.0723) -> (42.6059, 21.0723)
  line L94 (52.0197, 4.6887) -> (46.1777, 21.1987) construction
  line L95 (46.1777, 4.6887) -> (52.0197, 21.1987) construction
  line L96 (52.0197, 21.1987) -> (52.0197, 4.6887)
  line L97 (46.1777, 4.6887) -> (46.1777, 21.1987)
  line L98 (52.0197, 4.6887) -> (46.1777, 4.6887)
  line L99 (46.1777, 21.1987) -> (52.0197, 21.1987)
  line L100 (61.4336, 4.6887) -> (55.5916, 21.1987) construction
  line L101 (55.5916, 4.6887) -> (61.4336, 21.1987) construction
  line L102 (61.4336, 21.1987) -> (61.4336, 4.6887)
  line L103 (55.5916, 4.6887) -> (55.5916, 21.1987)
  line L104 (61.4336, 4.6887) -> (55.5916, 4.6887)
  line L105 (55.5916, 21.1987) -> (61.4336, 21.1987)
  line L106 (70.8405, 4.603) -> (64.9985, 21.113) construction
  line L107 (64.9985, 4.603) -> (70.8405, 21.113) construction
  line L108 (70.8405, 21.113) -> (70.8405, 4.603)
  line L109 (64.9985, 4.603) -> (64.9985, 21.113)
  line L110 (70.8405, 4.603) -> (64.9985, 4.603)
  line L111 (64.9985, 21.113) -> (70.8405, 21.113)
  line L112 (80.2666, 4.6718) -> (74.4246, 21.1818) construction
  line L113 (74.4246, 4.6718) -> (80.2666, 21.1818) construction
  line L114 (80.2666, 21.1818) -> (80.2666, 4.6718)
  line L115 (74.4246, 4.6718) -> (74.4246, 21.1818)
  line L116 (80.2666, 4.6718) -> (74.4246, 4.6718)
  line L117 (74.4246, 21.1818) -> (80.2666, 21.1818)
  line L118 (83.6994, 4.6188) -> (89.5414, 21.1288) construction
  line L119 (83.6994, 21.1288) -> (89.5414, 21.1288)
  line L120 (89.5414, 4.6188) -> (83.6994, 4.6188)
  line L121 (83.6994, 4.6188) -> (83.6994, 21.1288)
  line L122 (89.5414, 4.6188) -> (83.6994, 21.1288) construction
  line L123 (89.5414, 21.1288) -> (89.5414, 4.6188)
  line L124 (93.1333, 4.6718) -> (98.9753, 21.1818) construction
  line L125 (93.1333, 21.1818) -> (98.9753, 21.1818)
  line L126 (98.9753, 4.6718) -> (93.1333, 4.6718)
  line L127 (93.1333, 4.6718) -> (93.1333, 21.1818)
  line L128 (98.9753, 4.6718) -> (93.1333, 21.1818) construction
  line L129 (98.9753, 21.1818) -> (98.9753, 4.6718)
  line L130 (102.5141, 4.5128) -> (108.3561, 21.0228) construction
  line L131 (102.5141, 21.0228) -> (108.3561, 21.0228)
  line L132 (108.3561, 4.5128) -> (102.5141, 4.5128)
  line L133 (102.5141, 4.5128) -> (102.5141, 21.0228)
  line L134 (108.3561, 4.5128) -> (102.5141, 21.0228) construction
  line L135 (108.3561, 21.0228) -> (108.3561, 4.5128)
  line L136 (74.4246, 4.6718) -> (80.2666, 21.1818) construction
  line L137 (74.4246, 21.1818) -> (80.2666, 21.1818)
  line L138 (80.2666, 4.6718) -> (74.4246, 4.6718)
  line L139 (74.4246, 4.6718) -> (74.4246, 21.1818)
  line L140 (80.2666, 4.6718) -> (74.4246, 21.1818) construction
  line L141 (80.2666, 21.1818) -> (80.2666, 4.6718)
  point P0 (-8.4699, 13.0684)
  point P1 (1.5175, 13.1981)
  point P2 (11.5697, 13.1332)
  point P3 (-18.3401, 13.0684)
  point P4 (-28.3044, 13.1624)
  point P5 (-38.3925, 13.1038)
  point P6 (-48.4106, 13.1254)
  point P7 (-58.3958, 13.2966)
  point P8 (-68.381, 13.0113)
  point P9 (-78.3091, 13.0684)
  point P10 (21.0468, 13.0069)
  point P11 (30.367, 13.1332)
  point P12 (39.6849, 12.8173)
  point P13 (49.0987, 12.9437)
  point P14 (58.5126, 12.9437)
  point P15 (67.9195, 12.858)
  point P16 (77.3456, 12.9268)
  point P17 (86.6204, 12.8738)
  point P18 (96.0543, 12.9268)
  point P19 (105.4351, 12.7678)
  point P20 (77.3456, 12.9268)
  dimension "d72" = 5.842
  dimension "d73" = 16.51
  dimension "d74" = 5.842
  dimension "d75" = 16.51
  dimension "d76" = 5.842
  dimension "d77" = 16.51
  dimension "d78" = 5.842
  dimension "d79" = 16.51
  dimension "d80" = 5.842
  dimension "d81" = 16.51
  dimension "d82" = 5.842
  dimension "d83" = 16.51
  dimension "d84" = 5.842
  dimension "d85" = 16.51
  dimension "d86" = 5.842
  dimension "d87" = 16.51
  dimension "d88" = 5.842
  dimension "d89" = 16.51
  dimension "d90" = 5.842
  dimension "d91" = 16.51
  dimension "d92" = 5.842
  dimension "d93" = 16.51
  dimension "d94" = 5.842
  dimension "d95" = 16.51
  dimension "d96" = 5.842
  dimension "d97" = 16.51
  dimension "d98" = 5.842
  dimension "d99" = 16.51
  dimension "d100" = 5.842
  dimension "d101" = 16.51
  dimension "d102" = 5.842
  dimension "d103" = 16.51
  dimension "d104" = 5.842
  dimension "d105" = 16.51
  dimension "d106" = 5.842
  dimension "d107" = 16.51
  dimension "d108" = 5.842
  dimension "d109" = 16.51
  dimension "d110" = 5.842
  dimension "d111" = 16.51
  dimension "d112" = 5.842
  dimension "d113" = 16.51
  constraint horizontal L16
  constraint perpendicular L16 L17
  constraint parallel L16 L18
  constraint parallel L17 L19
  constraint coincident L20 P0
  constraint coincident L21 P0
  constraint horizontal L25
  constraint perpendicular L25 L26
  constraint parallel L25 L27
  constraint parallel L23 L26
  constraint coincident P1 L22
  constraint coincident P1 L24
  constraint horizontal L31
  constraint perpendicular L31 L32
  constraint parallel L31 L33
  constraint parallel L29 L32
  constraint coincident P2 L28
  constraint coincident P2 L30
  constraint horizontal L37
  constraint perpendicular L37 L38
  constraint parallel L37 L39
  constraint parallel L35 L38
  constraint coincident P3 L34
  constraint coincident P3 L36
  constraint horizontal L43
  constraint perpendicular L43 L44
  constraint parallel L43 L45
  constraint parallel L41 L44
  constraint coincident P4 L40
  constraint coincident P4 L42
  constraint horizontal L49
  constraint perpendicular L49 L50
  constraint parallel L49 L51
  constraint parallel L47 L50
  constraint coincident P5 L46
  constraint coincident P5 L48
  constraint horizontal L55
  constraint perpendicular L55 L56
  constraint parallel L55 L57
  constraint parallel L53 L56
  constraint coincident P6 L52
  constraint coincident P6 L54
  constraint horizontal L61
  constraint perpendicular L61 L62
  constraint parallel L61 L63
  constraint parallel L59 L62
  constraint coincident P7 L58
  constraint coincident P7 L60
  constraint horizontal L67
  constraint perpendicular L67 L68
  constraint parallel L67 L69
  constraint parallel L65 L68
  constraint coincident P8 L64
  constraint coincident P8 L66
  constraint horizontal L73
  constraint perpendicular L73 L74
  constraint parallel L73 L75
  constraint parallel L71 L74
  constraint coincident P9 L70
  constraint coincident P9 L72
  constraint horizontal L80
  constraint perpendicular L79 L80
  constraint parallel L80 L81
  constraint parallel L78 L79
  constraint coincident P10 L76
  constraint coincident P10 L77
  constraint horizontal L86
  constraint perpendicular L85 L86
  constraint parallel L86 L87
  constraint parallel L84 L85
  constraint coincident P11 L82
  constraint coincident P11 L83
  constraint horizontal L92
  constraint perpendicular L91 L92
  constraint parallel L92 L93
  constraint parallel L90 L91
  constraint coincident P12 L88
  constraint coincident P12 L89
  constraint horizontal L98
  constraint perpendicular L97 L98
  constraint parallel L98 L99
  constraint parallel L96 L97
  constraint coincident P13 L94
  constraint coincident P13 L95
  constraint horizontal L104
  constraint perpendicular L103 L104
  constraint parallel L104 L105
  constraint parallel L102 L103
  constraint coincident P14 L100
  constraint coincident P14 L101
  constraint horizontal L110
  constraint perpendicular L109 L110
  constraint parallel L110 L111
  constraint parallel L108 L109
  constraint coincident P15 L106
  constraint coincident P15 L107
  constraint horizontal L116
  constraint perpendicular L115 L116
  constraint parallel L116 L117
  constraint parallel L114 L115
  constraint coincident P20 L112
  constraint coincident P20 L113
  constraint horizontal L120
  constraint perpendicular L120 L121
  constraint parallel L119 L120
  constraint parallel L121 L123
  constraint coincident P17 L122
  constraint coincident P17 L118
  constraint horizontal L126
  constraint perpendicular L126 L127
  constraint parallel L125 L126
  constraint parallel L127 L129
  constraint coincident P18 L128
  constraint coincident P18 L124
  constraint horizontal L132
  constraint perpendicular L132 L133
  constraint parallel L131 L132
  constraint parallel L133 L135
  constraint coincident P19 L134
  constraint coincident P19 L130
  constraint horizontal L138
  constraint perpendicular L138 L139
  constraint parallel L137 L138
  constraint parallel L139 L141
  constraint coincident P20 L140
  constraint coincident P20 L136
  measures "d72" distance of L17.end L18.end
  measures "d73" distance of L16.end L17.end
  measures "d74" distance of L22.end L23.start
  measures "d75" distance of L24.start L22.end
  measures "d76" distance of L28.end L29.start
  measures "d77" distance of L30.start L28.end
  measures "d78" distance of L34.end L35.start
  measures "d79" distance of L36.start L34.end
  measures "d80" distance of L40.end L41.start
  measures "d81" distance of L42.start L40.end
  measures "d82" distance of L46.end L47.start
  measures "d83" distance of L48.start L46.end
  measures "d84" distance of L52.end L53.start
  measures "d85" distance of L54.start L52.end
  measures "d86" distance of L58.end L59.start
  measures "d87" distance of L60.start L58.end
  measures "d88" distance of L64.end L65.start
  measures "d89" distance of L66.start L64.end
  measures "d90" distance of L70.end L71.start
  measures "d91" distance of L72.start L70.end
  measures "d92" distance of L77.end L76.end
  measures "d93" distance of L77.start L76.end
  measures "d94" distance of L83.end L82.end
  measures "d95" distance of L83.start L82.end
  measures "d96" distance of L89.end L88.end
  measures "d97" distance of L89.start L88.end
  measures "d98" distance of L95.end L94.end
  measures "d99" distance of L95.start L94.end
  measures "d100" distance of L101.end L100.end
  measures "d101" distance of L101.start L100.end
  measures "d102" distance of L107.end L106.end
  measures "d103" distance of L107.start L106.end
  measures "d104" distance of L113.end L112.end
  measures "d105" distance of L113.start L112.end
  measures "d106" distance of L118.end L119.start
  measures "d107" distance of L118.start L119.start
  measures "d108" distance of L124.end L125.start
  measures "d109" distance of L124.start L125.start
  measures "d110" distance of L130.end L131.start
  measures "d111" distance of L130.start L131.start
  measures "d112" distance of L113.end L112.end
  measures "d113" distance of L113.start L112.end
extrude "Extrude12" cut sketch "Sketch16" against normal blind 38.1 contours L16 L17 L18 L19 | L23 L25 L26 L27 | L29 L31 L32 L33 | L35 L37 L38 L39 | L41 L43 L44 L45 | L47 L49 L50 L51 | L53 L55 L56 L57 | L59 L61 L62 L63 | L65 L67 L68 L69 | L71 L73 L74 L75 | L78 L79 L80 L81 | L84 L85 L86 L87 | L90 L91 L92 L93 | L96 L97 L98 L99 | L102 L103 L104 L105 | L108 L109 L110 L111 | L114 L115 L116 L117 L137 L138 L139 L141 | L119 L120 L121 L123 | L125 L126 L127 L129 | L131 L132 L133 L135 bodies 1
chamfer "Chamfer4" distance 4.699 angle 45 20 edges at (78.3091, -21.3234, 8.001) (68.381, -21.2663, 8.001) (58.3958, -21.5516, 8.001) (48.4106, -21.3804, 8.001) (38.3925, -21.3588, 8.001) (28.3044, -21.4174, 8.001) (18.3401, -21.3234, 8.001) (8.4699, -21.3234, 8.001) (-1.5175, -21.4531, 8.001) (-11.5697, -21.3882, 8.001) (-21.0468, -21.2619, 8.001) (-30.367, -21.3882, 8.001) (-39.6849, -21.0723, 8.001) (-49.0987, -21.1987, 8.001) (-58.5126, -21.1987, 8.001) (-67.9195, -21.113, 8.001) (-77.3456, -21.1818, 8.001) (-86.6204, -21.1288, 8.001) (-96.0543, -21.1818, 8.001) (-105.4351, -21.0228, 8.001) on bodies 1
chamfer "Chamfer5" distance 4.699 angle 45 20 edges at (78.3091, -4.8134, 8.001) (68.381, -4.7563, 8.001) (58.3958, -5.0416, 8.001) (48.4106, -4.8704, 8.001) (38.3925, -4.8488, 8.001) (28.3044, -4.9074, 8.001) (18.3401, -4.8134, 8.001) (8.4699, -4.8134, 8.001) (-1.5175, -4.9431, 8.001) (-11.5697, -4.8782, 8.001) (-21.0468, -4.7519, 8.001) (-30.367, -4.8782, 8.001) (-39.6849, -4.5623, 8.001) (-49.0987, -4.6887, 8.001) (-58.5126, -4.6887, 8.001) (-67.9195, -4.603, 8.001) (-77.3456, -4.6718, 8.001) (-86.6204, -4.6188, 8.001) (-96.0543, -4.6718, 8.001) (-105.4351, -4.5128, 8.001) on bodies 1
fillet "Fillet2" radius 2.032 4 edges at (0, -27.305, 8.001) (-152.4, 0, 8.001) (0, 27.305, 8.001) (152.4, 0, 8.001) on bodies 1
sketch "Sketch17" plane through (-152.4, 0, 0) normal (-1, 0, 0) x (0, -1, 0)
  line L0 (27.305, 5.969) -> (-27.305, 5.969)
  line L1 (-27.305, 5.969) -> (-27.305, 0)
  line L2 (-27.305, 0) -> (-24.6876, 0)
  line L3 (-24.6876, 0) -> (-24.6876, 2.7305)
  arc A0 (-23.4176, 4.0005) -> (-24.6876, 2.7305) centre (-23.4176, 2.7305) ccw
  line L4 (-23.4176, 4.0005) -> (-21.59, 4.0005)
  line L5 (-21.59, 4.0005) -> (-21.59, 0)
  line L6 (-21.59, 0) -> (22.225, 0)
  line L7 (22.225, 0) -> (22.225, -1.6256)
  line L8 (22.225, -1.6256) -> (19.685, -1.6256)
  line L9 (19.685, -1.6256) -> (19.685, -7.874)
  line L10 (19.685, -7.874) -> (27.305, -7.874)
  line L11 (27.305, -7.874) -> (27.305, 5.969)
  line L12 (22.225, 0) -> (-24.6451, 0)
  line L13 (-24.6451, 0) -> (-24.6451, -5.3044)
  line L14 (-24.6451, -5.3044) -> (22.225, -5.3044)
  line L15 (22.225, -5.3044) -> (22.225, 0)
  constraint horizontal L12
  constraint vertical L13
  constraint horizontal L14
  constraint vertical L15
  constraint coincident L6.end L7.start
extrude "Extrude13" cut sketch "Sketch17" against normal blind 335.28 contours L6 L7 L8 L9 L12 L13 L14 L15 | L8 L9 L14 L15 bodies 1 2 3 4
